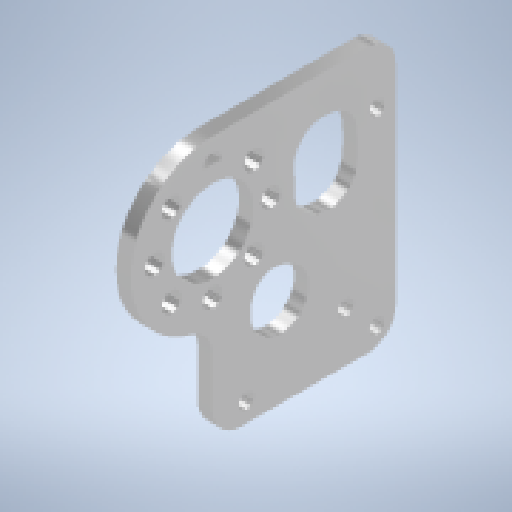
# Autodesk Inventor part: toe_joint
Saved by Autodesk Inventor 2024.1 (Build 281209000, 209)
## iProperties
Created: 2024-02-11
Part Number: toe_joint
Material: アルミニウム 6061
Document SubType Name: Modeling
Designer: hibik
Density: 2.7 g/cm^3
Appearance: アルミニウム - フラット
Author: hibik
Autodesk Inventor part; units mm, degrees
ref_plane "YZ Plane" through (0, 0, 0) normal (1, 0, 0) x (0, 1, 0)
ref_plane "XZ Plane" through (0, 0, 0) normal (0, 1, 0) x (-1, 0, 0)
ref_plane "XY Plane" through (0, 0, 0) normal (0, 0, 1) x (1, 0, 0)
sketch "スケッチ1" plane through (0, 0, 0) normal (1, 0, 0) x (0, 1, 0)
  circle A0 centre (0, 0) radius 4.25
  circle A1 centre (0, 0) radius 6
  circle A2 centre (6, 0) radius 1
  line L0 (-25.8, 0) -> (21.8, 0) projected
  circle A3 centre (4.2426, 4.2426) radius 1
  circle A4 centre (0, 6) radius 1
  circle A5 centre (-4.2426, 4.2426) radius 1
  circle A6 centre (-6, 0) radius 1
  circle A7 centre (-4.2426, -4.2426) radius 1
  line L1 (0, 8.5) -> (-19, 8.5)
  line L2 (-19, 8.5) -> (-19, -8.5)
  line L3 (-19, -8.5) -> (0, -8.5)
  circle A8 centre (0, 0) radius 8.5
  circle A9 centre (0, 0) radius 15
  line L4 (8.5, 0) -> (-19, 0)
  line L5 (-19, 0) -> (-19, -15)
  line L6 (-19, -15) -> (8.5, -15)
  line L7 (8.5, -15) -> (8.5, 0)
  line L8 (8.5, -15) -> (-19, -15)
  line L9 (-19, -15) -> (-19, -19)
  line L10 (-19, -19) -> (8.5, -19)
  line L11 (8.5, -19) -> (8.5, -15)
  line L12 (4.5, -7.2111) -> (4.5, -14.3091)
  line L13 (-14.4568, -4) -> (-7.5, -4)
  circle A10 centre (-17, -3.5) radius 0.8 projected
  circle A11 centre (-13.8033, -13.8033) radius 0.8 projected
  circle A12 centre (-17, -17) radius 0.8 projected
  circle A13 centre (2.5, -17) radius 0.8 projected
  line L14 (-1.7321, 1) -> (1.7321, -1)
  line L15 (1.7321, -1) -> (-6.2194, -14.7723)
  line L16 (-6.2194, -14.7723) -> (-9.6835, -12.7723)
  line L17 (-9.6835, -12.7723) -> (-1.7321, 1)
  circle A14 centre (0, -6) radius 1
  circle A15 centre (4.2426, -4.2426) radius 1
  point P0 (9.5, 0)
  point P1 (0, 8.5)
  point P2 (0, -8.5)
  point P3 (-8.5, 0)
  point P4 (-19, 0)
  point P5 (7, 0)
  point P6 (5.9167, -0.9965)
  point P7 (-3.4791, -4.8884)
  point P8 (-4.8884, -3.4791)
  point P9 (-5.9167, -0.9965)
  point P10 (-5.9167, 0.9965)
  point P11 (-4.8884, 3.4791)
  point P12 (-7, 0)
  point P13 (-3.4791, 4.8884)
  point P14 (-0.9965, 5.9167)
  point P15 (0.9965, 5.9167)
  point P16 (3.4791, 4.8884)
  point P17 (4.8884, 3.4791)
  point P18 (5.9167, 0.9965)
  point P19 (5, 0)
  point P20 (4.25, 0)
  point P21 (-4.25, 0)
  point P22 (-5, 0)
  point P23 (-19, 0)
  point P24 (-12.3592, 8.5)
  point P25 (-15, 0)
  point P26 (-9.1651, -11.8744)
  point P27 (-5.701, -13.8744)
  point P28 (-2.3986, -8.1545)
  point P29 (-5.8627, -6.1545)
  dimension "d1" = 12
  dimension "d0" = 8.5
  dimension "d2" = 2
  dimension "d5" = 360
  dimension "d7" = 17
  dimension "d12" = 19
  dimension "d13" = 30
  dimension "d14" = 4
  dimension "d18" = 4
  dimension "d19" = 4
  dimension "d20" = 4
  dimension "d21" = 30
  constraints: 34 end point, 11 centre point, 7 parallel, 7 point on circle, 6 coincident, 5 perpendicular, 4 point on line, 3 horizontal, 2 collinear, 2 midpoint, 2 tangent, 1 vertical, 20 other
  measures "d0" diameter of A0
  measures "d2" diameter of A2
  measures "d7" distance of L3.end L1.start
  measures "d12" distance from line of L2 point (0, 0)
  measures "d13" diameter of A9
  measures "d14" distance of L10.end L6.end
  measures "d18" distance between parallel lines of L0 L13
  measures "d19" distance between parallel lines of L7 L12
  measures "d20" distance between parallel lines of L17 L15
  measures "d21" angle of L8 L14
extrude "押し出し1" add sketch "スケッチ1" along normal blind 1.5 contours L0 A2 A1 A15 A14 L15 A0 | A0 L0 A6 A1 A5 A4 A3 A2 | A0 L17 A7 A1 A6 L0 | L15 A1 A7 L17 A0 | L0 A1 A2 | A2 A1 L0 | A14 A1 L15 | A1 A3 A4 A5 A6 L0 A8 A2 | A2 L0 A8 L15 A1 A14 A15 | A1 A7 L17 A8 L0 A6 | L15 A8 L17 A7 A1 | L15 L3 L17 A8 | L7 A9 L12 A8 | A8 L13 A9 L0 | L15 A9 L17 L3 | L7 L6 A9 | A9 L3 L2 L0 | L15 L16 L17 A9 | A9 L6 L5 L3 L17 L16 L15 | L11 L10 L9 L6 picked at (5.6738, -0.193) picked at (5.6738, 0.193)
fillet "フィレット1" radius 3 12 edges at (0.75, -8.5, 0) (0.75, -14.4568, -4) (0.75, -7.5, -4) (0.75, 4.5, -7.2111) (0.75, 4.5, -14.3091) (0.75, -19, 0) (0.75, -19, -19) (0.75, 8.5, -19) (0.75, -2.3986, -8.1545) (0.75, -5.8627, -6.1545) (0.75, -9.1651, -11.8744) (0.75, -5.701, -13.8744)
